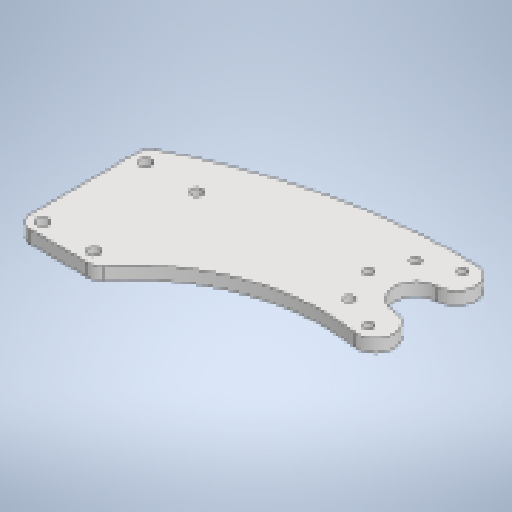
# Autodesk Inventor part: connectpart4
Saved by Autodesk Inventor 2024.3 (Build 283343010, 343A)
## iProperties
Created: 2025-06-28
Part Number: connectpart4
Material: アルミニウム 6061
Document SubType Name: Modeling
Designer: kshau
Density: 2.7 g/cm^3
Appearance: アルミニウム - フラット
Author: kshau
Autodesk Inventor part; units mm, degrees
ref_plane "YZ Plane" through (0, 0, 0) normal (1, 0, 0) x (0, 1, 0)
ref_plane "XZ Plane" through (0, 0, 0) normal (0, 1, 0) x (-1, 0, 0)
ref_plane "XY Plane" through (0, 0, 0) normal (0, 0, 1) x (1, 0, 0)
sketch "スケッチ1" plane through (0, 0, 0) normal (0, 1, 0) x (-1, 0, 0)
  circle A0 centre (0, 0) radius 5
  circle A1 centre (0, 0) radius 11
  line L0 (0, 0) -> (0, -11)
  line L1 (0, 0) -> (0, 11)
  circle A2 centre (0, 9.5) radius 4.5
  circle A3 centre (0, -9.5) radius 4.5
  circle A4 centre (2.3645, 112.8492) radius 126.872
  circle A5 centre (8.3362, 58.5776) radius 45.2805
  circle A6 centre (2.3645, 112.8492) radius 54.5992
  line L2 (62.25, 31) -> (44.25, 31)
  line L3 (44.25, 31) -> (44.25, 1)
  line L4 (44.25, 1) -> (62.25, 1)
  line L5 (62.25, 1) -> (62.25, 31)
  line L6 (0, 0) -> (13.75, 0)
  line L7 (13.75, 0) -> (13.75, -16.75)
  line L8 (13.75, -16.75) -> (0, -16.75)
  line L9 (0, -16.75) -> (0, 0)
  line L10 (70.25, 35.25) -> (36.25, 35.25)
  line L11 (36.25, 35.25) -> (36.25, -11.25)
  line L12 (36.25, -11.25) -> (70.25, -11.25)
  line L13 (70.25, -11.25) -> (70.25, 35.25)
  line L14 (70.25, 0) -> (36.25, 0)
  line L15 (0, 0) -> (36.25, 0)
  point P0 (62.25, 1)
  point P1 (0.7536, 13.9365)
  point P2 (0, 5)
  point P3 (0, -5)
  point P4 (-0.087, -13.9992)
  dimension "d4" = 253.744
  dimension "d5" = 90.561
  dimension "d0" = 10
  dimension "d1" = 22
  dimension "d2" = 9
  dimension "d3" = 9
  dimension "d7" = 18
  dimension "d8" = 30
  dimension "d9" = 13.75
  dimension "d10" = 16.75
  dimension "d11" = 46.5
  dimension "d12" = 4.25
  dimension "d13" = 8
  dimension "d14" = 34
  dimension "d15" = 11.25
  dimension "d16" = 70.25
  constraints: 32 end point, 6 parallel, 6 point on line, 5 coincident, 4 centre point, 4 perpendicular, 3 horizontal, 2 point on circle, 2 tangent, 1 vertical, 11 other
  measures "d0" diameter of A0
  measures "d1" diameter of A1
  measures "d2" diameter of A2
  measures "d3" diameter of A3
  measures "d7" distance between parallel lines of L3 L5
  measures "d8" distance of L4.end L2.start
  measures "d9" distance from line of A0.centre L7
  measures "d10" distance of L6.end L7.end
  measures "d11" distance of L12.end L10.start
  measures "d12" distance between parallel lines of L10 L2
  measures "d13" distance between parallel lines of L5 L13
  measures "d14" distance of L11.end L12.end
  measures "d15" distance between parallel lines of L12 L14
  measures "d16" distance from line of point (0, 0) L13
extrude "押し出し1" add sketch "スケッチ1" along normal blind 3 contours L6 A1 A3 A0 | A0 A2 A1 L6 | A2 A1 L1 | L1 A1 A2 | A3 A1 L0 | L0 A1 A3 | L6 L7 A4 A3 A1 | A1 A2 A5 L11 L15 L6 | A1 A2 | L9 A3 A1 | A1 A3 L9 | L15 L11 A4 L7 | L14 A4 L11 | L11 A5 L3 L4 A4 L14 | L2 L5 L4 L3
fillet "フィレット1" radius 3 3 edges at (-62.25, 1.5, 1) (-62.25, 1.5, 31) (-44.25, 1.5, 31)
sketch "スケッチ4" plane through (0, 3, 0) normal (0, 1, 0) x (1, 0, 0)
  arc A0 (0, 5) -> (0.087, 13.9992) centre (0, 9.5) ccw projected
  arc A1 (-0.7536, -13.9365) -> (0, -5) centre (0, -9.5) ccw projected
  arc A2 (0, 5) -> (0, -5) centre (0, 0) ccw projected
  circle A3 centre (0, 0) radius 11
  point P0 (0, 11)
  point P1 (0, -11)
  point P2 (-7.7782, -7.7782)
  point P3 (-11, 0)
  point P4 (-7.7782, 7.7782)
  point P5 (0, 11)
  dimension "d29" = 22
  dimension "d56" = 180
  constraints: 2 point on circle, 1 centre point, 1 coincident, 5 other
  measures "d29" diameter of A3
hole "穴1" at (0, 3, -11) at (0, 3, 11) at (-7.7782, 3, 7.7782) at (-11, 3, 0) at (-7.7782, 3, -7.7782) direction (0, -1, 0) diameter 2.2 end through all
sketch "スケッチ5" plane through (0, 3, 0) normal (0, 1, 0) x (1, 0, 0)
  line L0 (-59.25, -4) -> (-47.25, -4)
  line L1 (-47.25, -4) -> (-47.25, -28)
  line L2 (-47.25, -28) -> (-59.25, -28)
  line L3 (-59.25, -28) -> (-59.25, -4)
  line L4 (-62.25, -2.8114) -> (-62.25, -28) projected
  line L5 (-59.25, -31) -> (-45.6995, -31) projected
  point P0 (0, 0)
  dimension "d37" = 3
  dimension "d38" = 3
  dimension "d39" = 12
  dimension "d40" = 24
  constraints: 8 end point, 4 coincident, 2 parallel, 1 horizontal, 1 perpendicular
  measures "d37" distance between parallel lines of L4 L3
  measures "d38" distance between parallel lines of L5 L2
  measures "d39" distance of L1.end L2.end
  measures "d40" distance of L0.end L1.end
hole "穴2" at (-59.25, 3, 28) at (-47.25, 3, 28) at (-47.25, 3, 4) at (-59.25, 3, 4) direction (0, -1, 0) diameter 2.7 end through all
